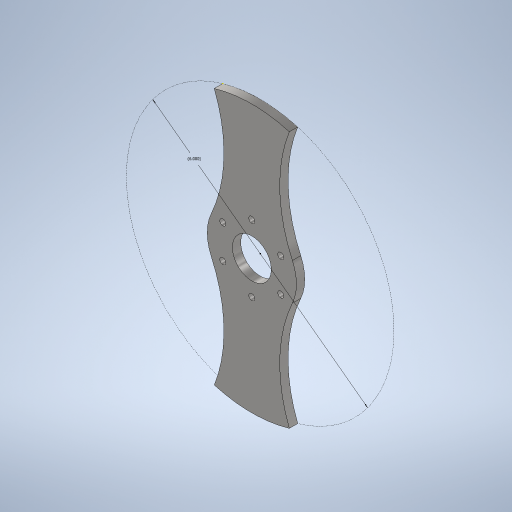
# Autodesk Inventor part: Blade (Bar)
Saved by Autodesk Inventor 2023.4 (Build 274418000, 418)
## iProperties
Created: 2022-06-12
Part Number: Blade (Bar)
Material: Stainless Steel
Document SubType Name: Modeling
Designer: Nathan Cai
Density: 8 g/cm^3
Appearance: Semi-Polished
Mass: 209.485 g
Surface Area: 133.7 cm^2
Volume: 26.1856 cm^3
Author: Nathan Cai
Autodesk Inventor part; units mm, degrees
ref_plane "YZ Plane" through (0, 0, 0) normal (1, 0, 0) x (0, 1, 0)
ref_plane "XZ Plane" through (0, 0, 0) normal (0, 1, 0) x (-1, 0, 0)
ref_plane "XY Plane" through (0, 0, 0) normal (0, 0, 1) x (1, 0, 0)
sketch "Sketch1" plane through (0, 0, 0) normal (0, 0, 1) x (1, 0, 0)
  circle A0 centre (0, 0) radius 11.1125
  line L0 (0, 0) -> (0, 19.05) construction
  circle A1 centre (0, 19.05) radius 1.7526
  circle A2 centre (-16.4978, 9.525) radius 1.7526
  circle A3 centre (-16.4978, -9.525) radius 1.7526
  circle A4 centre (0, -19.05) radius 1.7526
  circle A5 centre (16.4978, -9.525) radius 1.7526
  circle A6 centre (16.4978, 9.525) radius 1.7526
  circle A7 centre (0, 0) radius 76.2 construction
  line L1 (-15.875, -74.528) -> (15.875, -74.528) construction
  line L2 (15.875, -74.528) -> (15.875, 74.528) construction
  line L3 (15.875, 74.528) -> (-15.875, 74.528) construction
  line L4 (-15.875, 74.528) -> (-15.875, -74.528) construction
  line L5 (-15.875, -74.528) -> (15.875, 74.528) construction
  line L6 (15.875, -74.528) -> (-15.875, 74.528) construction
  line L7 (0, 76.2) -> (0, -76.2) construction
  line L8 (0, 0) -> (21.3699, 73.1421) construction
  circle A8 centre (0, 0) radius 66.675 construction
  circle A9 centre (0, 0) radius 25.4
  line L9 (21.3699, 73.1421) -> (17.8969, 64.2282) construction
  arc A10 (21.3699, 73.1421) -> (-21.3699, 73.1421) centre (0, 0) ccw
  line L10 (-15.875, 0) -> (15.875, 0) construction
  arc A11 (-21.3699, -73.1421) -> (21.3699, -73.1421) centre (0, 0) ccw
  arc A12 (21.3699, 73.1421) -> (23.1163, 10.5259) centre (96.4161, 43.9028) ccw
  arc A13 (-23.1163, 10.5259) -> (-21.3699, 73.1421) centre (-96.4161, 43.9028) ccw
  arc A14 (23.1163, -10.5259) -> (21.3699, -73.1421) centre (96.4161, -43.9028) ccw
  arc A15 (-21.3699, -73.1421) -> (-23.1163, -10.5259) centre (-96.4161, -43.9028) ccw
  point P0 (0, 74.528)
  point P1 (0, -66.675)
  point P2 (23.1163, -10.5259)
  point P3 (-23.1163, -10.5259)
  point P4 (-23.1163, 10.5259)
  dimension "d10" = 50.8
  dimension "d0" = 22.225
  dimension "d1" = 19.05
  dimension "d2" = 3.5052
  dimension "d5" = 360
  dimension "d7" = 152.4
  dimension "d8" = 31.75
  dimension "d9" = 9.525
  dimension "d11" = 5
  constraints: 22 end point, 19 point on circle, 15 centre point, 9 symmetric about line, 7 midpoint, 4 coincident, 2 parallel, 2 perpendicular, 2 tangent, 1 horizontal, 1 point on line, 1 vertical, 22 other
  measures "d0" diameter of A0
  measures "d1" distance of L0.start L0.end
  measures "d2" diameter of A1
  measures "d7" diameter of A7
  measures "d8" distance of L3.end L2.end
  measures "d9" radial gap between concentric circles of A7 A8
  measures "d11" angle of L9 L8
extrude "Extrusion1" add sketch "Sketch1" along normal blind 4.7625
sketch "Sketch3" plane through (0, 0, 0) normal (0, 0, -1) x (-1, 0, 0)
  circle A0 centre (0, 0) radius 76.2 construction
  point P0 (21.3699, 73.1421)
  dimension "d25" = 152.4
  constraints: 1 coincident, 3 other
body "Solid1"
